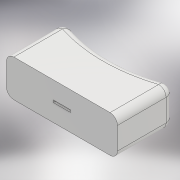
# Autodesk Inventor part: pot slider
Saved by Autodesk Inventor 2017 (Build 210142000, 142)
## iProperties
Created: 2017-03-04
Part Number: pot slider
Material: ABS Plastic
Document SubType Name: Modeling
Designer: dpgai
Density: 1.06 g/cm^3
Appearance: Smooth - White
Author: dpgai
Autodesk Inventor part; units mm, degrees
ref_plane "YZ Plane" through (0, 0, 0) normal (1, 0, 0) x (0, 1, 0)
ref_plane "XZ Plane" through (0, 0, 0) normal (0, 1, 0) x (-1, 0, 0)
sketch "Sketch1" plane through (0, 0, 0) normal (0, 0, 1) x (1, 0, 0)
  line L0 (0, 0) -> (0, 12)
  line L1 (15, 0) -> (-15, 0)
  line L2 (-15, 0) -> (-15, 12)
  line L3 (-15, 12) -> (15, 12)
  line L4 (15, 12) -> (15, 0)
  line L5 (-15, 12) -> (-15, 16)
  line L6 (15, 12) -> (15, 16)
  arc A0 (-15, 16) -> (15, 16) centre (0, 53.081) ccw
  point P0 (0, 12)
  dimension "d0" = 12
  dimension "d1" = 30
  dimension "d2" = 4
  dimension "d3" = 4
  dimension "d4" = 40
  constraints: 14 end point, 3 vertical, 2 parallel, 2 point on circle, 1 centre point, 1 coincident, 1 horizontal, 1 midpoint, 1 perpendicular
  measures "d0" distance of L0.start L0.end
  measures "d1" distance of L2.end L3.end
  measures "d2" distance of L2.end L5.end
  measures "d3" distance of L3.end L6.end
  measures "d4" radius of A0
extrude "Extrusion1" add sketch "Sketch1" along normal blind 10
fillet "Fillet1" radius 2 8 edges at (-15, 16, 5) (15, 16, 5) (0, 13.081, 10) (0, 13.081, 0) (15, 8, 10) (-15, 8, 10) (15, 8, 0) (-15, 8, 0)
ref_plane "Work Plane1" through (0, 0, 5) normal (0, 0, 1) x (1, 0, 0)
sketch "Sketch2" plane through (0, 0, 5) normal (0, 0, 1) x (1, 0, 0)
  line L0 (-13, 0) -> (13, 0) projected
  line L1 (-2.5, 0) -> (2.5, 0)
  line L2 (-1.6, 15) -> (1.6, 15)
  line L3 (-1.6, 15) -> (-2.5, 0)
  line L4 (1.6, 15) -> (2.5, 0)
  line L5 (-2.32, 3) -> (2.32, 3)
  line L6 (-2.32, 0) -> (2.32, 0)
  line L7 (-1.6, 12) -> (1.6, 12)
  line L8 (-1.6, 12) -> (-2.32, 0)
  line L9 (2.32, 0) -> (1.6, 12)
  point P0 (0, 0)
  point P1 (0, 0)
  point P2 (0, 15)
  point P3 (0, 0)
  point P4 (0, 12)
  dimension "d9" = 5
  dimension "d10" = 2.5
  dimension "d11" = 3.2
  dimension "d13" = 12
  dimension "d14" = 4.64
  dimension "d15" = 4.64
  dimension "d16" = 2.32
  dimension "d17" = 3.2
  dimension "d18" = 12
  constraints: 18 end point, 6 point on line, 3 horizontal, 3 midpoint, 2 vertical alignment, 1 coincident
  measures "d9" distance of L1.start L1.end
  measures "d10" distance of point (0, 0) L1.start
  measures "d11" distance of L2.start L2.end
  measures "d13" distance between parallel lines of L2 L5
  measures "d14" distance of L5.start L5.end
  measures "d15" distance of L6.start L6.end
  measures "d16" distance of point (0, 0) L6.end
  measures "d17" distance of L7.start L7.end
  measures "d18" distance between parallel lines of L0 L7
extrude "Extrusion2" cut sketch "Sketch2" along normal mid plane 0.6 contours L8 L5 L9 L0 | L8 L7 L9 L5
body "Solid1"
